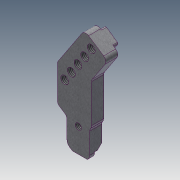
# Autodesk Inventor part: J005048
Saved by Autodesk Inventor 2015 SP1 (Build 190203100, 203)
## iProperties
Created: 2014-10-30
Material: STAINLESS STEEL, 303
Vendor: HHMI: JFRC - ID&F
Document SubType Name: Modeling
Designer: arnoldj
Density: 8 g/cm^3
Mass: 37.2011 g
Surface Area: 34.3864 cm^2
Volume: 4.65014 cm^3
Description: MBS INLINE CLAMP ARM
Project: P-201804
Appearance: Metal-Steel (Stainless, Brushed)
Part Number: J005048
RuleStatus: InUse
AfterDocSave0: file://Part Number Cleaner
LAB/DEPT: SVOBODA (LAB)
REQUESTING SCIENTIST: SOFRONIEW, NICK
SURFACE ROUGHNESS: 63 Ra
DESIGN DEPARTMENT: HHMI: JRC - ID&F
SPECIAL FINISH: NONE
ALTERED ITEM PART NUMBER: N/A
ALTERED ITEM VENDOR: N/A
ALTERED ITEM DESCRIPTION: N/A
Revision Number: A
Autodesk Inventor part; units mm, degrees
ref_plane "YZ Plane" through (0, 0, 0) normal (1, 0, 0) x (0, 1, 0)
ref_plane "XZ Plane" through (0, 0, 0) normal (0, 1, 0) x (-1, 0, 0)
ref_plane "XY Plane" through (0, 0, 0) normal (0, 0, 1) x (1, 0, 0)
sketch "Sketch1" plane through (0, 0, 0) normal (0, 0, 1) x (1, 0, 0)
  line L0 (-6, 18.161) -> (6, 18.161)
  line L1 (6, 18.161) -> (6, 0)
  line L2 (6, 0) -> (-6, 0)
  line L3 (-6, 0) -> (-6, 18.161)
  line L4 (0, 70.590027) -> (0, -11.765004)
  line L5 (-14.474625, 0) -> (9.412437, 0)
  point P0 (0, 0)
  point P1 (0, 0)
  point P2 (0, 18.161)
  dimension "d0" = 12
  dimension "d1" = 18.161
  constraints: 8 end point, 2 midpoint, 2 parallel, 2 vertical alignment, 1 horizontal, 1 horizontal alignment, 1 perpendicular
  measures "d0" distance of L0.start L0.end
  measures "d1" distance of L2.end L0.start
extrude "Extrusion1" add sketch "Sketch1" along normal blind 2.54
chamfer "Chamfer2" distance 2.54 angle 45 1 edges at (6, 0, 1.27)
chamfer "Chamfer23" distance 3.175 angle 56.5 1 edges at (-6, 0, 1.27) measured on face at (-6, 6.0537, 1.6933)
chamfer "Chamfer5" distance 1.27 angle 45 1 edges at (1.1285, 0, 2.54)
fillet "Fillet4" radius 3.175 4 edges at (3.46, 0, 0.635) (6, 2.54, 1.27) (-6, 3.175, 1.27) (-1.2031, 0, 0.635)
sketch "Sketch32" plane through (0, 0, 0) normal (0, 0, -1) x (-1, 0, 0)
  line L0 (6, 18.161) -> (5.0292, 18.161)
  line L1 (5.0292, 18.161) -> (5.0292, 4.4958)
  line L2 (5.0292, 4.4958) -> (6, 4.4958)
  line L3 (6, 4.4958) -> (6, 18.161)
  line L4 (-6, 18.161) -> (-5.0292, 18.161)
  line L5 (-5.0292, 18.161) -> (-5.0292, 3.855128)
  line L6 (-6, 3.855128) -> (-6, 18.161)
  line L7 (0, -11.765004) -> (0, 70.590027)
  line L8 (-9.412437, 0) -> (14.474625, 0)
  line L9 (-6, 3.855128) -> (-5.0292, 3.855128)
  point P0 (0, 0)
  point P1 (-5.0292, 4.4958)
  dimension "d353" = 13.6652
  dimension "d356" = 10.0584
  dimension "d361" = 14.30587
  constraints: 16 end point, 3 horizontal, 3 parallel, 3 point on line, 2 perpendicular, 1 other
  measures "d353" distance of L2.end L0.start
  measures "d356" distance between parallel lines of L5 L1
  measures "d361" distance of L4.end L5.end
sketch "Sketch34" plane through (0, 0, 0) normal (0, 0, 1) x (1, 0, 0)
  line L0 (0, 70.590027) -> (0, -11.765004)
  line L1 (-13.986592, 0) -> (6.484243, 0)
  circle A0 centre (0, 5.3848) radius 1.5875
  point P0 (0, 0)
  dimension "d346" = 3.175
  dimension "d347" = 5.3848
  constraints: 1 centre point, 1 point on line
  measures "d346" diameter of A0
  measures "d347" distance from line of L1 A0.centre
extrude "Extrusion25" add sketch "Sketch34" against normal blind 1.143
chamfer "Chamfer24" distance 0.127 angle 45 1 edges at (-1.5875, 5.3848, -1.143)
extrude "Extrusion26" add sketch "Sketch32" along normal blind 3.81
chamfer "Chamfer25" distance 2.54 angle 45 2 edges at (-5.5146, 4.4958, -3.81) (5.5146, 3.8551, -3.81)
fillet "Fillet40" radius 0.254 4 edges at (6, 3.8551, -0.635) (-5.0292, 4.4958, -0.635) (-6, 4.4958, -0.635) (5.0292, 3.8551, -0.635)
sketch "Sketch9" plane through (0, 0, 2.54) normal (0, 0, 1) x (1, 0, 0)
  line L0 (-6, 18.161) -> (6, 18.161)
  line L1 (-6, 4.880989) -> (-6, 18.161)
  line L2 (0, 70.590027) -> (0, -11.765004)
  line L3 (7.016, 38.735853) -> (7.016, 17.156009)
  line L4 (-16.481679, 0) -> (21.454761, 0)
  line L5 (7.016, 38.735853) -> (15.42752, 51.444273)
  line L6 (11.767105, 55.624156) -> (0, 37.846) construction
  line L7 (-11.062187, 37.884046) -> (3.248617, 59.505313)
  line L8 (15.42752, 51.444273) -> (3.248617, 59.505313)
  line L9 (-11.062187, 18.971589) -> (-6, 15.621)
  line L10 (-6, 4.880989) -> (-6, 18.161)
  line L11 (7.016, 17.156009) -> (6, 15.621)
  line L12 (6, 18.161) -> (6, 3.855128)
  line L13 (6, 18.161) -> (6, 3.855128)
  line L14 (-6, 15.621) -> (6, 15.621) construction
  line L15 (-6, 18.161) -> (6, 18.161)
  line L16 (6, 18.161) -> (6, 15.621)
  line L17 (-6, 18.161) -> (-6, 15.621)
  line L18 (-11.062187, 18.971589) -> (-11.062187, 37.884046)
  point P0 (-6.5, 3.855128)
  point P1 (0, 0)
  point P2 (-6, 6.731)
  point P3 (-6, 11.811)
  point P4 (6, 11.811)
  point P5 (6, 6.731)
  dimension "d154" = 146.5
  dimension "d188" = 19.685
  dimension "d243" = 9.2456
  dimension "d244" = 5.3594
  dimension "d265" = 2.54
  dimension "d343" = 1.016
  dimension "d383" = 6.0706
  dimension "d384" = 56.5
  dimension "d466" = 15.24
  constraints: 24 end point, 3 parallel, 3 point on line, 2 collinear, 2 perpendicular, 2 vertical, 4 other
  measures "d154" angle of L5 L3
  measures "d188" distance from line of L0 L6.end
  measures "d243" distance between parallel lines of L6 L7
  measures "d244" distance between parallel lines of L6 L5
  measures "d265" distance from line of L0 L9.end
  measures "d343" distance between parallel lines of L3 L12
  measures "d383" distance of L9.start L9.end
  measures "d384" angle to the sketch y axis of L9
  measures "d466" distance of L3.start L5.end
extrude "Extrusion6-Main Body" add sketch "Sketch9" against normal blind 6.35
sketch "Sketch37" plane through (0, 0, -3.81) normal (0, 0, -1) x (-1, 0, 0)
  line L0 (-15.42752, 51.444273) -> (-3.248617, 59.505313)
  line L1 (-5.366687, 58.103393) -> (-12.250415, 53.547153)
  line L2 (-12.250415, 53.547153) -> (11.062187, 18.325654)
  line L3 (11.062187, 37.884046) -> (11.062187, 18.971589)
  line L4 (11.062187, 33.282071) -> (11.062187, 18.325654)
  line L5 (11.062187, 37.884046) -> (11.062187, 18.971589)
  line L6 (11.062187, 33.282071) -> (-5.366687, 58.103393)
  line L7 (-15.42752, 51.444273) -> (-3.248617, 59.505313)
  line L8 (-7.016, 38.735853) -> (-15.42752, 51.444273)
  point P0 (0, 0)
  dimension "d420" = 8.255
  dimension "d465" = 3.81
  constraints: 8 end point, 4 point on line, 2 perpendicular, 1 collinear
  measures "d420" distance between parallel lines of L2 L6
  measures "d465" distance between parallel lines of L8 L2
extrude "Extrusion29" add sketch "Sketch37" along normal blind 2.54
sketch "Sketch38" plane through (0, 0, -6.35) normal (0, 0, -1) x (-1, 0, 0)
  line L0 (-8.808551, 55.825273) -> (11.062187, 25.803862) construction
  line L1 (-3.248617, 59.505313) -> (11.062187, 37.884046) construction
  line L2 (7.20398, 31.632977) -> (12.763914, 35.313017) construction
  line L3 (-3.310419, 47.518502) -> (2.249514, 51.198542) construction
  line L4 (0.194381, 42.223327) -> (5.754314, 45.903367) construction
  line L5 (3.69918, 36.928152) -> (9.259114, 40.608192) construction
  circle A0 centre (-3.310419, 47.518502) radius 2.5 construction
  circle A1 centre (7.20398, 31.632977) radius 2.5 construction
  line L6 (-4.690262, 49.603217) -> (-5.937187, 48.777895) construction
  line L7 (-12.250415, 53.547153) -> (11.062187, 18.325654)
  line L8 (11.062187, 33.282071) -> (-5.366687, 58.103393)
  line L9 (-5.366687, 58.103393) -> (-12.250415, 53.547153)
  line L10 (11.062187, 18.325654) -> (11.062187, 33.282071)
  line L11 (-6.815219, 52.813677) -> (-1.255285, 56.493717) construction
  line L12 (-3.248617, 59.505313) -> (11.062187, 37.884046) construction
  line L13 (-5.366687, 58.103393) -> (-3.248617, 59.505313)
  line L14 (-21.065806, 0) -> (18.402201, 0)
  point P0 (0, 0)
  point P1 (-3.559838, 58.825022)
  dimension "d415" = 5
  dimension "d407" = 6.35
  dimension "d410" = 6.35
  dimension "d411" = 6.35
  dimension "d412" = 9.96152
  dimension "d413" = 6.9903
  dimension "d416" = 5
  dimension "d421" = 8.255
  dimension "d422" = 4.1275
  dimension "d427" = 6.35
  dimension "d461" = 19.6903
  dimension "d464" = 42.22333
  constraints: 14 end point, 7 point on line, 2 coincident, 2 midpoint, 1 centre point, 1 parallel, 1 perpendicular, 15 other
  measures "d407" distance between parallel lines of L3 L4
  measures "d410" distance between parallel lines of L4 L5
  measures "d411" distance between parallel lines of L2 L5
  measures "d412" distance from line of L0.start L3
  measures "d413" distance from line of L0.end L2
  measures "d416" diameter of A1
  measures "d421" distance between parallel lines of L7 L8
  measures "d422" distance between parallel lines of L7 L0
  measures "d427" distance from line of L3 L11.start
  measures "d461" distance from line of L0.end L4
  measures "d464" distance from line of L4.start L14
hole "Hole3" at (-0.194381, 42.223327, -6.35) at (-3.69918, 36.928152, -6.35) at (3.310419, 47.518502, -6.35) at (6.815219, 52.813677, -6.35) at (-7.20398, 31.632977, -6.35) direction (0, 0, 1) diameter 4.1402 end through all
fillet "Fillet46" radius 0.635 4 edges at (-11.0622, 18.3257, -5.08) (5.3667, 58.1034, -5.08) (12.2504, 53.5472, -5.08) (-11.0622, 33.2821, -5.08)
fillet "Fillet47" radius 2.54 6 edges at (-6, 15.621, -0.635) (-11.0622, 18.9716, -0.635) (-11.0622, 37.884, -0.635) (3.2486, 59.5053, -0.635) (15.4275, 51.4443, -0.635) (7.016, 38.7359, -0.635)
fillet "Fillet48" radius 2.54 2 edges at (7.016, 17.156, -0.635) (6, 15.621, -0.635)
sketch "Sketch39" plane through (0, 0, -3.81) normal (0, 0, -1) x (-1, 0, 0)
  line L0 (5.0292, 18.161) -> (-5.0292, 18.161)
  line L1 (5.0292, 18.161) -> (-5.0292, 18.161)
  line L2 (-5.0292, 18.161) -> (-5.0292, 23.876)
  line L3 (-5.0292, 23.876) -> (5.0292, 23.876)
  line L4 (5.0292, 23.876) -> (5.0292, 18.161)
  line L5 (5.0292, 18.161) -> (-5.0292, 18.161)
  line L6 (0, -11.705065) -> (0, 70.230388)
  line L7 (-19.549473, 0) -> (16.164131, 0)
  point P0 (0, 0)
  dimension "d429" = 5.715
  dimension "d433" = 18.161
  dimension "d434" = 5.0292
  dimension "d435" = 10.0584
  constraints: 12 end point, 3 equal length, 1 perpendicular
  measures "d429" distance of L3.end L0.start
  measures "d433" distance between parallel lines of L7 L0
  measures "d434" distance between parallel lines of L6 L4
  measures "d435" distance of L2.end L3.end
extrude "Extrusion30" cut sketch "Sketch39" against normal blind 3.81
sketch "Sketch41" plane through (0, 0, 0) normal (0, 0, -1) x (-1, 0, 0)
  line L0 (5.0292, 23.876) -> (-5.0292, 23.876)
  line L1 (-5.0292, 23.876) -> (-5.0292, 10.795)
  line L2 (-5.0292, 10.795) -> (5.0292, 10.795)
  line L3 (5.0292, 10.795) -> (5.0292, 23.876)
  line L4 (-5.0292, 23.876) -> (-5.0292, 4.109128)
  point P0 (0, 0)
  dimension "d439" = 10.795
  constraints: 8 end point, 2 parallel, 2 perpendicular
  measures "d439" distance from line of L2 point (0, 0)
extrude "Extrusion31" add sketch "Sketch41" along normal blind 0.635
fillet "Fillet49" radius 1.651 4 edges at (-5.0292, 23.876, -2.2225) (5.0292, 23.876, -2.2225) (-5.0292, 10.795, -0.3175) (5.0292, 10.795, -0.3175)
sketch "Sketch42" plane through (0, 0, -3.81) normal (0, 0, -1) x (-1, 0, 0)
  point P0 (0, 0)
sketch "Sketch43" plane through (0, 0, -3.81) normal (0, 0, -1) x (-1, 0, 0)
  line L0 (0, -11.705065) -> (0, 70.230388)
  line L1 (-19.549473, 0) -> (16.164131, 0)
  line L2 (-3.3782, 23.876) -> (3.3782, 23.876)
  point P0 (0, 0)
  point P1 (0, 13.97)
  dimension "d450" = 13.97
  dimension "d458" = 9.906
  dimension "d459" = 23.876
  constraints: 1 point on line
  measures "d450" distance from line of L1 point (0, 13.97)
  measures "d458" distance from line of point (0, 13.97) L2
  measures "d459" distance from line of point (0, 0) L2
hole "Hole5" at (0, 13.97, -3.81) direction (0, 0, 1) diameter 3.2512 end through all
body "Solid1"
